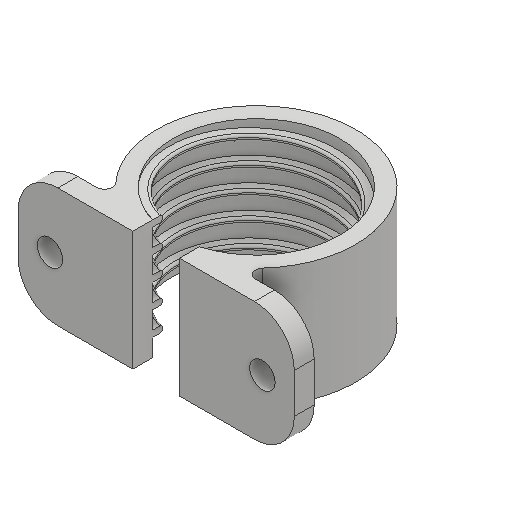
# Autodesk Inventor part: 3DP_ABS_Cable_Pipe_Mount
Saved by Autodesk Inventor 2026.1 (Build 301233000, 233)
## iProperties
Created: 2016-02-06
Part Number: 3DP_ABS_Cable_Pipe_Mount
Material: Ogólny
Document SubType Name: Modeling
Designer: Andrzej
Density: 1 g/cm^3
Appearance: Domyślna
Mass: 2.85351 g
Surface Area: 29.8559 cm^2
Volume: 2.85351 cm^3
Author: Andrzej
Autodesk Inventor part; units mm, degrees
ref_plane "YZ Plane" through (0, 0, 0) normal (1, 0, 0) x (0, 1, 0)
ref_plane "XZ Plane" through (0, 0, 0) normal (0, 1, 0) x (-1, 0, 0)
ref_plane "XY Plane" through (0, 0, 0) normal (0, 0, 1) x (1, 0, 0)
sketch "Szkic1" plane through (0, 0, 0) normal (0, 0, 1) x (1, 0, 0)
  arc A0 (2.9316, -4) -> (-2.9316, -4) centre (0, 6.0824) ccw
  arc A1 (7.3888, -4) -> (-7.3888, -4) centre (0, 6.0824) ccw
  line L0 (-17.3491, -4) -> (-17.3491, -6.5)
  line L1 (17.35, -6.5) -> (17.35, -4)
  line L2 (-2.9316, -4) -> (-2.9316, -6.5736)
  line L3 (2.9316, -4) -> (2.9316, -6.5)
  line L4 (-17.3491, -4) -> (-2.9316, -4)
  line L5 (2.9316, -4) -> (17.35, -4)
  line L6 (-17.3491, -6.5) -> (-2.9316, -6.5)
  line L7 (2.9316, -6.5) -> (17.35, -6.5)
  point P0 (0, 0)
  point P1 (-13.3491, -6.5736)
  point P2 (13.35, -6.4176)
  point P3 (0, -6.4176)
  dimension "d0" = 21
  dimension "d1" = 2
  dimension "d2" = 13.35
  dimension "d3" = 13.35
  dimension "d6" = 4
  dimension "d7" = 4
  dimension "d8" = 0
  constraints: 16 end point, 8 perpendicular, 5 point on circle, 3 point on line, 2 centre point, 2 horizontal, 1 vertical
  measures "d0" diameter of A0
  measures "d1" radial gap between concentric circles of A0 A1
  measures "d2" distance of point (-13.349, -6.574) point (0, -6.418)
  measures "d3" distance of point (0, -6.418) point (13.35, -6.418)
  measures "d6" distance from line of L1 point (13.35, -6.418)
  measures "d7" distance from line of point (-13.349, -6.574) L0
  measures "d8" horizontal distance of point (0, 0) point (0, -6.418)
extrude "Wyciągnięcie proste1" add sketch "Szkic1" along normal blind 15
fillet "Zaokrąglenie1" radius 1 2 edges at (7.3888, -4, 7.5) (-7.3888, -4, 7.5)
sketch "Szkic2" plane through (-17.3491, -6.5, 0) normal (0, -1, 0) x (1, 0, 0)
  line L0 (0, 0) -> (14.4174, 0) projected
  line L1 (14.4174, 0) -> (14.4174, 15) projected
  line L2 (0, 15) -> (14.4174, 15) projected
  line L3 (0, 0) -> (0, 15) projected
  line L4 (20.2807, 0) -> (34.6991, 0) projected
  line L5 (34.6991, 0) -> (34.6991, 15) projected
  line L6 (20.2807, 15) -> (34.6991, 15) projected
  line L7 (20.2807, 0) -> (20.2807, 15) projected
  line L8 (14.4174, 0) -> (14.4174, 15) projected
  line L9 (14.4174, 15) -> (20.2807, 15)
  line L10 (6.8491, 15) -> (27.8491, 15) projected
  line L11 (14.4174, 0) -> (20.2807, 0)
  line L12 (6.8491, 0) -> (27.8491, 0) projected
  point P0 (17.3491, 0)
  point P1 (3.9995, 7.5)
  point P2 (30.6995, 7.5)
  dimension "d12" = 15
  dimension "d13" = 7.5
  dimension "d14" = 7.5
  dimension "d15" = 26.7
  dimension "d16" = 34.6991
  dimension "d17" = 3.9995
  constraints: 4 end point, 2 collinear
  measures "d12" distance of L0.start L2.start
  measures "d13" distance from line of L2 point (4, 7.5)
  measures "d14" distance from line of L6 point (30.7, 7.5)
  measures "d15" distance of point (30.7, 7.5) point (4, 7.5)
  measures "d16" distance between parallel lines of L5 L3
  measures "d17" distance from line of L3 point (4, 7.5)
hole "Otwór1" at (-13.3495, -6.5, 7.5) at (13.3505, -6.5, 7.5) direction (0, 1, 0) diameter 3.2 depth 3
fillet "Zaokrąglenie2" radius 5 4 edges at (17.35, -5.25, 15) (17.35, -5.25, 0) (-17.3491, -5.25, 15) (-17.3491, -5.25, 0)
sketch "Szkic3" plane through (-2.9316, -6.5, 0) normal (1, 0, 0) x (0, 0, -1)
  line L0 (-10, 0) -> (-15, 0) projected
  line L1 (-5, 2.5) -> (0, 2.5) projected
  line L2 (-15, 0) -> (0, 0)
  line L3 (0, 0) -> (0, 2.5)
  line L4 (0, 2.5) -> (-15, 2.5)
  line L5 (-15, 2.5) -> (-15, 0)
  line L6 (-15, 2.5) -> (-14.2, 2.5)
  line L7 (-14.2, 2.5) -> (-14.2, 3.4)
  line L8 (-14.5, 3.7) -> (-14.7, 3.7)
  line L9 (-15, 3.4) -> (-15, 2.5)
  arc A0 (-14.7, 3.7) -> (-15, 3.4) centre (-14.7, 3.4) ccw
  arc A1 (-14.2, 3.4) -> (-14.5, 3.7) centre (-14.5, 3.4) ccw
  point P0 (0, 6.5)
  point P1 (-14.2, 3.7)
  point P2 (-15, 3.7)
  dimension "d26" = 0.8
  dimension "d27" = 1.2
  dimension "d36" = 0.3
  constraints: 16 end point, 4 parallel, 4 point on circle, 4 point on line, 4 tangent, 2 centre point, 2 horizontal, 2 perpendicular, 1 equal radius
  measures "d26" distance of point (-15, 3.7) point (-14.2, 3.7)
  measures "d27" distance of point (-14.2, 3.7) L6.end
  measures "d36" radius of A0
extrude "Wyciągnięcie proste2" cut sketch "Szkic2" against normal blind 5 contours L1 L9 L7 L11
coil "Zwój2" sketch "Szkic3" operation add axis through (0, 6.0824, 0) along (0, 0, -1) pitch 3 turns 4.7 hand right contours L9 A0 L8 A1 L7 L4
sketch "Szkic4" plane through (-2.9316, -6.5, 0) normal (0, -1, 0) x (1, 0, 0)
  arc A0 (15.2816, 0) -> (20.2816, 5) centre (15.2816, 5) ccw projected
  line L0 (20.2816, 5) -> (20.2816, 10) projected
  arc A1 (20.2816, 10) -> (15.2816, 15) centre (15.2816, 10) ccw projected
  line L1 (5.8633, 15) -> (15.2816, 15) projected
  line L2 (5.8633, 0) -> (5.8633, 15) projected
  line L3 (5.8633, 0) -> (15.2816, 0) projected
  circle A2 centre (16.2821, 7.5) radius 1.6 projected
  arc A3 (-14.4174, 5) -> (-9.4174, 0) centre (-9.4174, 5) ccw projected
  line L4 (-9.4174, 0) -> (0, 0) projected
  line L5 (0, 0) -> (0, 15) projected
  line L6 (-9.4174, 15) -> (0, 15) projected
  arc A4 (-9.4174, 15) -> (-14.4174, 10) centre (-9.4174, 10) ccw projected
  line L7 (-14.4174, 5) -> (-14.4174, 10) projected
  circle A5 centre (-10.4179, 7.5) radius 1.6 projected
  line L8 (-7.5684, 0) -> (13.4316, 0) projected
  line L9 (-7.5684, 15) -> (13.4316, 15) projected
  point P0 (2.9316, 0)
extrude "Wyciągnięcie proste3" cut sketch "Szkic4" against normal blind 10 contours L8 L5 L9 L2
equation "\"d3\" = d2"
equation "\"d13\" = 0.5 * d12"
equation "\"d14\" = d13"
equation "\"d17\" = -0.5 * d15 + 0.5 * d16"
